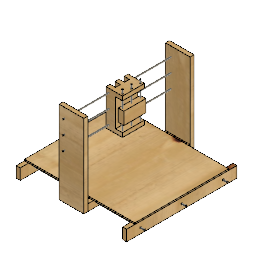
CNC_CAS_IEEE v10 (Autodesk Fusion 360 design; units mm, degrees)
Autodesk Fusion 360 part; units mm, degrees
sketch "Sketch1" plane through (0, 0, 0) normal (0, 0, 1) x (1, 0, 0)
  line L0 (-200, 200) -> (-200, -200)
  line L1 (200, -200) -> (200, 200)
  line L2 (200, 200) -> (-200, -200) construction
  line L3 (-200, 200) -> (200, -200) construction
  line L4 (-185, 185) -> (-185, -185)
  line L5 (185, -185) -> (185, 185)
  line L6 (185, -185) -> (185, -200)
  line L7 (185, -200) -> (200, -200)
  line L8 (-200, -200) -> (-185, -200)
  line L9 (-185, -200) -> (-185, -185)
  line L10 (-200, 200) -> (-185, 200)
  line L11 (-185, 200) -> (-185, 185)
  line L12 (185, 185) -> (185, 200)
  line L13 (185, 200) -> (200, 200)
  dimension "d1" = 400
  dimension "d2" = 400
  constraint parallel L0 L1
  constraint coincident L2 origin
  constraint coincident L3 origin
  constraint parallel L0 L4
  constraint parallel L1 L5
  constraint perpendicular L1 L7
  constraint perpendicular L0 L8
  constraint perpendicular L0 L10
  measures "d1" distance of L0.end L1.start
  measures "d2" distance of L0.start L0.end
extrude "Extrude1" add sketch "Sketch1" along normal blind 40 makes body 1 at (-185, 66.6667, 13.3333) makes body 2 at (185, 66.6667, 13.3333)
sketch "Sketch2" plane through (200, 0, 0) normal (1, 0, 0) x (0, 1, 0)
  line L0 (-200, 0) -> (200, 0)
  line L1 (200, 0) -> (200, 40)
  line L2 (200, 40) -> (-200, 40)
  line L3 (-200, 40) -> (-200, 0)
  circle A0 centre (-150, 20) radius 3
  circle A1 centre (150, 20) radius 3
  circle A2 centre (0, 20) radius 3
  dimension "d6" = 6
  dimension "d7" = 6
  dimension "d8" = 50
  dimension "d9" = 50
  dimension "d10" = 6
  dimension "d29" = 20
  constraint horizontal A0.centre A1.centre
  constraint horizontal A1.centre A2.centre
  measures "d6" diameter of A0
  measures "d7" diameter of A1
  measures "d8" distance of L1 A1.centre
  measures "d9" distance of L3 A0.centre
  measures "d10" diameter of A2
  measures "d29" distance of origin A2.centre
extrude "Extrude2" add sketch "Sketch2" against normal blind 415 separate body contours A0 | A1 | A2 makes body 3 at (-76.6667, -151.2575, 17.2763) makes body 4 at (-76.6667, 2.9876, 19.7272) makes body 5 at (-76.6667, 150.8749, 22.8696)
extrude "Extrude3" add sketch "Sketch2" along normal blind 15 separate body contours A0 | A1 | A2 makes body 6 at (210, -149.1875, 22.8879) makes body 7 at (210, 2.9851, 19.7013) makes body 8 at (210, 150.8125, 22.8879)
ref_plane "WorkPlane1" through (0, 0, 10) normal (0, 0, 1) x (1, 0, 0)
sketch "Sketch3" plane through (0, 0, 10) normal (0, 0, 1) x (1, 0, 0)
  line L0 (7.5, 170) -> (-7.5, 170)
  line L1 (-7.5, 170) -> (-7.5, -170)
  line L2 (-7.5, -170) -> (7.5, -170)
  line L3 (7.5, -170) -> (7.5, 170)
  line L4 (7.5, 170) -> (-7.5, -170) construction
  line L5 (-7.5, 170) -> (7.5, -170) construction
  line L6 (0, -170) -> (45, -170)
  line L7 (45, -170) -> (45, -185)
  line L8 (45, -185) -> (0, -185)
  line L9 (0, -185) -> (0, -170)
  line L10 (0, -170) -> (-45, -170)
  line L11 (-45, -170) -> (-45, -185)
  line L12 (-45, -185) -> (0, -185)
  line L13 (0, -185) -> (0, -170)
  line L14 (45, -170) -> (30, -170)
  line L15 (30, -170) -> (30, -125)
  line L16 (30, -125) -> (45, -125)
  line L17 (45, -125) -> (45, -170)
  line L18 (-45, -170) -> (-30, -170)
  line L19 (-30, -170) -> (-30, -125)
  line L20 (-30, -125) -> (-45, -125)
  line L21 (-45, -125) -> (-45, -170)
  line L22 (-100, 0) -> (80, 0) construction
  line L23 (30, 125) -> (45, 125)
  line L24 (30, 170) -> (30, 125)
  line L25 (45, 170) -> (30, 170)
  line L26 (45, 125) -> (45, 170)
  line L27 (45, 170) -> (45, 185)
  line L28 (0, 170) -> (45, 170)
  line L29 (45, 185) -> (0, 185)
  line L30 (-45, 170) -> (-45, 185)
  line L31 (-30, 125) -> (-45, 125)
  line L32 (-30, 170) -> (-30, 125)
  line L33 (-45, 170) -> (-30, 170)
  line L34 (-45, 185) -> (0, 185)
  line L35 (0, 170) -> (-45, 170)
  line L36 (-45, 125) -> (-45, 170)
  dimension "d16" = 340
  dimension "d17" = 15
  dimension "d18" = 45
  dimension "d19" = 15
  dimension "d20" = 45
  dimension "d21" = 15
  dimension "d22" = 15
  dimension "d23" = 45
  dimension "d24" = 22.5
  dimension "d25" = 45
  dimension "d26" = 15
  constraint perpendicular L0 L1
  constraint parallel L0 L2
  constraint parallel L1 L3
  constraint horizontal L0
  constraint coincident L4 origin
  constraint coincident L5 origin
  constraint horizontal L6
  constraint vertical L7
  constraint horizontal L8
  constraint vertical L9
  constraint midpoint L2 L6.start
  constraint horizontal L10
  constraint vertical L11
  constraint horizontal L12
  constraint vertical L13
  constraint horizontal L14
  constraint vertical L15
  constraint horizontal L16
  constraint vertical L17
  constraint horizontal L18
  constraint vertical L19
  constraint horizontal L20
  constraint vertical L21
  constraint perpendicular L3 L22
  constraint symmetric L6.start L22 L28.start
  constraint symmetric L6.end L22 L25.start
  constraint symmetric L7.end L22 L27.end
  constraint symmetric L8.end L22 L29.end
  constraint symmetric L10.end L22 L30.start
  constraint symmetric L11.end L22 L30.end
  constraint symmetric L14.end L22 L24.start
  constraint symmetric L15.end L22 L23.start
  constraint symmetric L16.end L22 L23.end
  constraint symmetric L18.end L22 L32.start
  constraint symmetric L19.end L22 L31.start
  constraint symmetric L20.end L22 L31.end
  measures "d16" distance of L0.end L1.end
  measures "d17" distance of L1.end L2.end
  measures "d18" distance of L6.start L6.end
  measures "d19" distance of L6.start L8.end
  measures "d20" distance of L6.start L10.end
  measures "d21" distance of L6.start L8.end
  measures "d22" distance of L6.end L14.end
  measures "d23" distance of L6.end L16.end
  measures "d24" distance of L2.end L14.end
  measures "d25" distance of L10.end L20.end
  measures "d26" distance of L10.end L18.end
extrude "Extrude4" add sketch "Sketch3" along normal blind 25 separate body makes body 9
ref_plane "WorkPlane2" through (0, 0, 40) normal (0, 0, 1) x (1, 0, 0)
sketch "Sketch4" plane through (0, 0, 40) normal (0, 0, 1) x (1, 0, 0)
  line L0 (-200, 200) -> (200, 200)
  line L1 (200, 200) -> (200, -200)
  line L2 (200, -200) -> (-200, -200)
  line L3 (-200, -200) -> (-200, 200)
  line L4 (-200, 170) -> (200, 170)
  line L5 (200, 170) -> (200, -170)
  line L6 (200, -170) -> (-200, -170)
  line L7 (-200, -170) -> (-200, 170)
  point P0 (-200, 200)
  point P1 (200, -200)
  constraint horizontal L0
  constraint vertical L1
  constraint horizontal L2
  constraint vertical L3
  constraint coincident P1 L1.end
  constraint coincident P0 L0.start
  constraint horizontal L4
  constraint vertical L5
  constraint horizontal L6
  constraint vertical L7
  constraint coincident L1 L5.end
  constraint coincident L3 L4.start
extrude "Extrude7" add sketch "Sketch4" along normal blind 5 separate body contours L1 L3 L4 L5 L6 L7 makes body 10
copy_body "Body->Comp1" bodies 1 removing the originals makes body 11 in component "base1"
copy_body "CutPasteBodies1" bodies 2 removing the originals makes body 12 in component "base1"
copy_body "CutPasteBodies2" bodies 3 4 5 removing the originals makes body 13 makes body 14 makes body 15 in component "base1"
copy_body "CutPasteBodies3" bodies 6 7 8 removing the originals makes body 16 makes body 17 makes body 18 in component "base1"
copy_body "Body->Comp2" bodies 9 removing the originals makes body 19 in component "carro1"
copy_body "Body->Comp3" bodies 10 removing the originals makes body 20 in component "tampa"
sketch "Sketch5" plane through (0, -185, 0) normal (0, -1, 0) x (1, 0, 0)
  line L0 (-45, 10) -> (45, 10)
  line L1 (45, 10) -> (45, 35)
  line L2 (45, 35) -> (-45, 35)
  line L3 (-45, 35) -> (-45, 10)
  line L4 (-45, 10) -> (45, 10)
  line L5 (45, 10) -> (45, 310)
  line L6 (45, 310) -> (-45, 310)
  line L7 (-45, 310) -> (-45, 10)
  circle A0 centre (-25, 275) radius 3
  circle A1 centre (-25, 225) radius 3
  circle A2 centre (-25, 175) radius 3
  line L8 (0, 275) -> (0, 310) construction
  dimension "d37" = 90
  dimension "d38" = 300
  dimension "d39" = 90
  dimension "d48" = 6
  dimension "d49" = 6
  dimension "d50" = 50
  dimension "d51" = 6
  dimension "d52" = 50
  dimension "d66" = 20
  dimension "d67" = 90
  dimension "d68" = 25
  constraint horizontal L4
  constraint vertical L5
  constraint horizontal L6
  constraint vertical L7
  constraint coincident L0.start L3.end
  constraint vertical A1.centre A2.centre
  constraint midpoint L6 L8.end
  constraint perpendicular L6 L8
  measures "d37" distance of L0.start L0.end
  measures "d38" distance of L0.start L6.end
  measures "d39" distance of L0.start L0.end
  measures "d48" diameter of A0
  measures "d49" diameter of A1
  measures "d50" distance of A0.centre A1.centre
  measures "d51" diameter of A2
  measures "d52" distance of A1.centre A2.centre
  measures "d66" distance of L7 A0.centre
  measures "d67" distance of L5.end L6.end
  measures "d68" distance of A0.centre L8.start
sketch "Sketch6" plane through (0, 185, 0) normal (0, 1, 0) x (-1, 0, 0)
  line L0 (-45, 10) -> (45, 10)
  line L1 (45, 10) -> (45, 35)
  line L2 (45, 35) -> (-45, 35)
  line L3 (-45, 35) -> (-45, 10)
  line L4 (-45, 10) -> (45, 10)
  line L5 (45, 10) -> (45, 310)
  line L6 (45, 310) -> (-45, 310)
  line L7 (-45, 310) -> (-45, 10)
  dimension "d42" = 300
  dimension "d43" = 90
  constraint horizontal L4
  constraint vertical L5
  constraint horizontal L6
  constraint vertical L7
  constraint coincident L0.start L3.end
  measures "d42" distance of L0.start L6.end
  measures "d43" distance of L0.start L0.end
extrude "Extrude1'" add sketch "Sketch5" along normal blind 15 separate body contours L0 L1 L2 L3 L4 L5 L7 | L2 L5 L6 L7 | A0 | A1 | A2 makes body 21 in component "carro1"
extrude "Extrude2'" add sketch "Sketch6" along normal blind 15 separate body makes body 22 in component "carro1"
extrude "Extrude8" add sketch "Sketch5" against normal blind 400 separate body contours A0 | A1 | A2 makes body 23 at (-26.9284, 81.6667, 177.2981) makes body 24 at (-26.9284, 81.6667, 227.2981) makes body 25 at (-27.4575, -51.6667, 273.2793)
extrude "Extrude9" add sketch "Sketch5" along normal blind 20 contours A0 | A1 | A2 bodies 23 24 25
copy_body "CutPasteBodies1'" bodies 23 24 25 removing the originals makes body 26 makes body 27 makes body 28 in component "carro1"
ref_plane "WorkPlane3" through (-22.0002, -47.9371, 224.9642) normal (0.999929, 0, -0.011947) x (0.011947, 0, 0.999929)
ref_plane "WorkPlane4" through (-25, 0, 0) normal (1, 0, 0) x (0, 1, 0)
sketch "Sketch9" plane through (-25, 0, 0) normal (1, 0, 0) x (0, 1, 0)
  line L0 (40.1014, 289.9773) -> (-39.8986, 289.9773) construction
  line L1 (-39.8986, 289.9773) -> (-39.8986, 159.9773) construction
  line L2 (-39.8986, 159.9773) -> (40.1014, 159.9773) construction
  line L3 (40.1014, 159.9773) -> (40.1014, 289.9773) construction
  line L4 (40.1014, 289.9773) -> (-39.8986, 159.9773) construction
  line L5 (-39.8986, 289.9773) -> (40.1014, 159.9773) construction
  line L6 (-39.8986, 159.9773) -> (-24.8986, 159.9773)
  line L7 (-24.8986, 159.9773) -> (-24.8986, 289.9773)
  line L8 (-24.8986, 289.9773) -> (-39.8986, 289.9773)
  line L9 (-39.8986, 289.9773) -> (-39.8986, 159.9773)
  line L10 (7.6014, 289.9773) -> (-7.3986, 289.9773)
  line L11 (-7.3986, 289.9773) -> (-7.3986, 159.9773)
  line L12 (-7.3986, 159.9773) -> (7.6014, 159.9773)
  line L13 (7.6014, 159.9773) -> (7.6014, 289.9773)
  line L14 (7.6014, 289.9773) -> (-7.3986, 159.9773) construction
  line L15 (-7.3986, 289.9773) -> (7.6014, 159.9773) construction
  line L16 (40.1014, 159.9773) -> (25.1014, 159.9773)
  line L17 (25.1014, 159.9773) -> (25.1014, 289.9773)
  line L18 (25.1014, 289.9773) -> (40.1014, 289.9773)
  line L19 (40.1014, 289.9773) -> (40.1014, 159.9773)
  point P0 (0.1014, 224.9773)
  point P1 (0.1014, 224.9773)
  dimension "d70" = 80
  dimension "d71" = 130
  dimension "d72" = 15
  dimension "d73" = 130
  dimension "d74" = 15
  dimension "d75" = 130
  dimension "d76" = 130
  dimension "d77" = 15
  constraint perpendicular L0 L1
  constraint parallel L0 L2
  constraint parallel L1 L3
  constraint horizontal L0
  constraint coincident L4 P1
  constraint coincident L5 P1
  constraint horizontal L6
  constraint vertical L7
  constraint horizontal L8
  constraint vertical L9
  constraint perpendicular L10 L11
  constraint parallel L10 L12
  constraint parallel L11 L13
  constraint horizontal L10
  constraint coincident L14 P1
  constraint coincident L15 P1
  constraint coincident P1 P0
  constraint horizontal L16
  constraint vertical L17
  constraint horizontal L18
  constraint vertical L19
  measures "d70" distance of L1.end L2.end
  measures "d71" distance of L0.end L1.end
  measures "d72" distance of L1.end L6.end
  measures "d73" distance of L1.end L0.end
  measures "d74" distance of L11.end L12.end
  measures "d75" distance of L10.end L11.end
  measures "d76" distance of L2.end L0.start
  measures "d77" distance of L2.end L16.end
extrude "Extrude10" add sketch "Sketch9" along normal blind 10 separate body makes body 29 at (-25, -34.8986, 246.644) makes body 30 at (-25, -2.3986, 246.644) makes body 31 at (-25, 35.1014, 203.3107)
extrude "Extrude11" add 3 faces at (-25, 35.1014, 203.3107) (-25, -2.3986, 246.644) (-25, -34.8986, 246.644) along direction (-1, 0, 0) blind 10 on bodies 29 30 31 bodies 31 29 30
sketch "Sketch10" plane through (-15, 0, 0) normal (1, 0, 0) x (0, 1, 0)
  line L0 (7.6014, 159.9773) -> (7.6014, 289.9773)
  line L1 (7.6014, 289.9773) -> (-7.3986, 289.9773)
  line L2 (-7.3986, 289.9773) -> (-7.3986, 159.9773)
  line L3 (-7.3986, 159.9773) -> (7.6014, 159.9773)
  line L4 (-39.8986, 289.9773) -> (40.1014, 289.9773)
  line L5 (40.1014, 289.9773) -> (40.1014, 159.9773)
  line L6 (40.1014, 159.9773) -> (-39.8986, 159.9773)
  line L7 (-39.8986, 159.9773) -> (-39.8986, 289.9773)
  point P0 (-39.8986, 289.9773)
  point P1 (40.1014, 159.9773)
  constraint horizontal L4
  constraint vertical L5
  constraint horizontal L6
  constraint vertical L7
  constraint coincident P1 L5.end
  constraint coincident P0 L4.start
extrude "Extrude12" add sketch "Sketch10" along normal blind 15 bodies 29 30 31
sketch "Sketch11" plane through (0, 0, 0) normal (1, 0, 0) x (0, 1, 0)
  line L0 (-39.8986, 159.9773) -> (40.1014, 159.9773)
  line L1 (40.1014, 159.9773) -> (40.1014, 289.9773)
  line L2 (40.1014, 289.9773) -> (-39.8986, 289.9773)
  line L3 (-39.8986, 289.9773) -> (-39.8986, 159.9773)
  line L4 (-39.8986, 289.9773) -> (40.1014, 289.9773)
  line L5 (40.1014, 289.9773) -> (40.1014, 274.9773)
  line L6 (40.1014, 274.9773) -> (-39.8986, 274.9773)
  line L7 (-39.8986, 274.9773) -> (-39.8986, 289.9773)
  line L8 (40.1014, 289.9773) -> (25.1014, 289.9773)
  line L9 (25.1014, 274.9773) -> (40.1014, 274.9773)
  line L10 (40.1014, 274.9773) -> (40.1014, 289.9773)
  line L11 (-39.8986, 159.9773) -> (-24.8986, 159.9773)
  line L12 (-24.8986, 159.9773) -> (-24.8986, 174.9773)
  line L13 (-24.8986, 174.9773) -> (-39.8986, 174.9773)
  line L14 (-39.8986, 174.9773) -> (-39.8986, 159.9773)
  line L15 (40.1014, 159.9773) -> (25.1014, 159.9773)
  line L16 (25.1014, 159.9773) -> (25.1014, 174.9773)
  line L17 (25.1014, 174.9773) -> (40.1014, 174.9773)
  line L18 (40.1014, 174.9773) -> (40.1014, 159.9773)
  line L19 (-24.8986, 274.9773) -> (-24.8986, 289.9773)
  line L20 (25.1014, 274.9773) -> (25.1014, 289.9773)
  line L21 (-24.8986, 174.9773) -> (25.1014, 174.9773)
  point P0 (-24.8986, 289.9773)
  dimension "d84" = 80
  dimension "d85" = 15
  dimension "d86" = 15
  dimension "d87" = 15
  dimension "d88" = 15
  dimension "d89" = 15
  dimension "d90" = 15
  dimension "d91" = 15
  constraint horizontal L4
  constraint vertical L5
  constraint horizontal L6
  constraint vertical L7
  constraint coincident L2.end L3.start
  constraint horizontal L8
  constraint horizontal L9
  constraint vertical L10
  constraint coincident L1.end L2.start
  constraint horizontal L11
  constraint vertical L12
  constraint horizontal L13
  constraint vertical L14
  constraint coincident L0.start L3.end
  constraint horizontal L15
  constraint vertical L16
  constraint horizontal L17
  constraint vertical L18
  constraint coincident L0.end L1.start
  constraint coincident L6 L19.start
  constraint coincident P0 L19.end
  constraint perpendicular L4 L19
  constraint perpendicular L4 L20
  measures "d84" distance of L2.end L1.end
  measures "d85" distance of L2.end L6.end
  measures "d86" distance of L1.end L8.end
  measures "d87" distance of L1.end L5.end
  measures "d88" distance of L0.start L11.end
  measures "d89" distance of L0.start L13.end
  measures "d90" distance of L0.end L15.end
  measures "d91" distance of L0.end L17.end
extrude "Extrude13" add sketch "Sketch11" along normal blind 25 contours L0 L3 L11 L12 L13 L14 | L0 L12 L16 L21 | L0 L1 L15 L16 L17 L18 | L2 L3 L4 L6 L7 L19 | L2 L4 L6 L19 L20 | L1 L2 L4 L5 L6 L8 L9 L10 L20 bodies 29
sketch "Sketch12" plane through (0, 0, 289.9773) normal (0, 0, 1) x (-1, 0, 0)
  line L0 (35, 39.8986) -> (-25, 39.8986)
  line L1 (-25, 39.8986) -> (-25, -40.1014)
  line L2 (-25, -40.1014) -> (35, -40.1014)
  line L3 (35, -40.1014) -> (35, -25.1014)
  line L4 (35, -25.1014) -> (15, -25.1014)
  line L5 (15, -25.1014) -> (15, -7.6014)
  line L6 (15, -7.6014) -> (35, -7.6014)
  line L7 (35, -7.6014) -> (35, 7.3986)
  line L8 (35, 7.3986) -> (15, 7.3986)
  line L9 (15, 7.3986) -> (15, 24.8986)
  line L10 (15, 24.8986) -> (35, 24.8986)
  line L11 (35, 24.8986) -> (35, 39.8986)
  circle A0 centre (-17.5, 32.3986) radius 2.5
  circle A1 centre (-17.5, -32.6014) radius 2.5
  circle A2 centre (-17.5, -0.1014) radius 2.5
  dimension "d94" = 5
  dimension "d95" = 5
  dimension "d96" = 7.5
  dimension "d97" = 7.5
  dimension "d98" = 7.5
  dimension "d99" = 7.5
  dimension "d100" = 5
  dimension "d101" = 40
  constraint vertical A1.centre A2.centre
  measures "d94" diameter of A0
  measures "d95" diameter of A1
  measures "d96" distance of L2 A1.centre
  measures "d97" distance of L1 A1.centre
  measures "d98" distance of L1 A0.centre
  measures "d99" distance of L0 A0.centre
  measures "d100" diameter of A2
  measures "d101" distance of L0 A2.centre
extrude "Extrude14" add sketch "Sketch12" against normal blind 135 separate body contours A0 | A1 | A2 makes body 32 at (15.0124, -32.1497, 244.9773) makes body 33 at (15.0124, 0.3503, 244.9773) makes body 34 at (15.0124, 32.8503, 244.9773)
extrude "Extrude15" add 3 faces at (16.8022, 32.0078, 289.9773) (16.8115, 0.3551, 289.9773) (18.324, -32.5228, 289.9773) along direction (0, 0, 1) blind 14 separate body on bodies 32 33 34 makes body 35 at (15.0124, 0.3503, 299.3107) makes body 36 at (15.0124, 32.8503, 299.3107) makes body 37 at (15.0124, -32.1497, 299.3107)
sketch "Sketch13" plane through (0, 40.1014, 0) normal (0, 1, 0) x (-1, 0, 0)
  line L0 (35, 289.9773) -> (-25, 289.9773)
  line L1 (-25, 289.9773) -> (-25, 274.9773)
  line L2 (-25, 274.9773) -> (0, 274.9773)
  line L3 (0, 274.9773) -> (0, 174.9773)
  line L4 (0, 174.9773) -> (-25, 174.9773)
  line L5 (-25, 174.9773) -> (-25, 159.9773)
  line L6 (-25, 159.9773) -> (35, 159.9773)
  line L7 (35, 159.9773) -> (35, 289.9773)
  line L8 (-10, 200) -> (-30, 200)
  line L9 (-30, 200) -> (-30, 215)
  line L10 (-30, 215) -> (-10, 215)
  line L11 (-10, 215) -> (-10, 200)
  line L12 (-10, 230) -> (-30, 230)
  line L13 (-30, 230) -> (-30, 245)
  line L14 (-30, 245) -> (-10, 245)
  line L15 (-10, 245) -> (-10, 230)
  line L16 (-10, 215) -> (-10, 230)
  line L17 (-30, 215) -> (-30, 230)
  dimension "d107" = 20
  dimension "d108" = 15
  dimension "d109" = 20
  dimension "d110" = 15
  constraint horizontal L8
  constraint vertical L9
  constraint horizontal L10
  constraint vertical L11
  constraint horizontal L12
  constraint vertical L13
  constraint horizontal L14
  constraint vertical L15
  constraint perpendicular L12 L16
  measures "d107" distance of L8.start L8.end
  measures "d108" distance of L8.start L10.end
  measures "d109" distance of L12.start L12.end
  measures "d110" distance of L12.start L14.end
extrude "Extrude16" add sketch "Sketch13" against normal blind 80 separate body contours L8 L9 L10 L11 | L10 L12 L16 L17 | L12 L13 L14 L15 makes body 38
copy_body "Body->Comp4" bodies 29 removing the originals makes body 39 in component "carro2"
copy_body "CutPasteBodies1''" bodies 32 33 34 35 36 37 removing the originals makes body 40 makes body 41 makes body 42 makes body 43 makes body 44 makes body 45 in component "carro2"
copy_body "Body->Comp5" bodies 38 removing the originals makes body 46 in component "carro3"
component "base1" placed x (1, 0, 0) y (0, 1, 0) z (0, 0, 1) at (0, 0, 0)
component "carro1" placed x (1, 0, 0) y (0, 1, 0) z (0, 0, 1) at (0, 0, 0)
component "tampa" placed x (1, 0, 0) y (0, 1, 0) z (0, 0, 1) at (0, 0, 0)
component "carro2" placed x (1, 0, 0) y (0, 1, 0) z (0, 0, 1) at (0, 0, 0)
component "carro3" placed x (1, 0, 0) y (0, 1, 0) z (0, 0, 1) at (0, 0, 0)
equation "d98 = d97"
equation "d99 = d96"
named bodies: "base1", "carro1"
